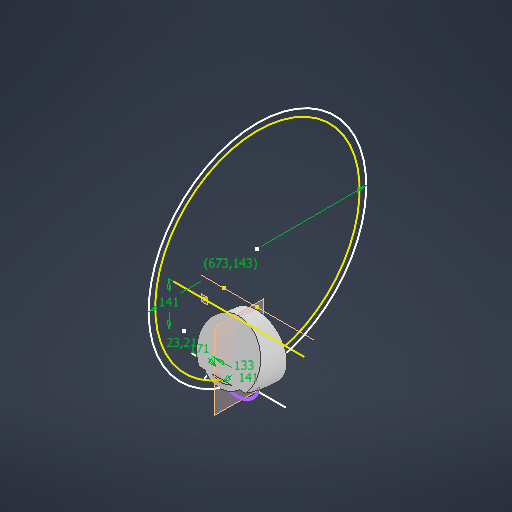
# Autodesk Inventor part: направление мяча 2
Saved by Autodesk Inventor 2026.2 (Build 302298000, 298)
## iProperties
Created: 2025-11-28
Part Number: направление мяча 2
Material: Типовые
Document SubType Name: Modeling
Designer: Phantom
Density: 1 g/cm^3
Appearance: По умолчанию
Author: Phantom
Autodesk Inventor part; units mm, degrees
ref_plane "XZ Plane" through (0, 0, 0) normal (0, 1, 0) x (-1, 0, 0)
sketch "Эскиз1" plane through (0, 0, 0) normal (0, 0, 1) x (1, 0, 0)
  arc A0 (72.3251, -161) -> (129.6749, -161) centre (101, -101) ccw
  arc A1 (47.332, -161) -> (154.668, -161) centre (101, -101) ccw
  line L0 (-97.5257, 0) -> (307.6841, 0) projected
  line L1 (-39.6386, -161) -> (244.9538, -161)
  line L2 (101, -167.5) -> (101, -181.5)
  arc A2 (171.1424, -161) -> (30.8576, -161) centre (101, -101) ccw
  arc A3 (169.1564, -161) -> (32.8436, -161) centre (101, -101) ccw
  arc A4 (173.1049, -161) -> (28.8951, -161) centre (101, -101) ccw
  line L3 (188.8611, -125.2269) -> (188.512, -125.2269)
  line L4 (188.512, -125.2269) -> (191.6745, -125.0262)
  line L5 (13.488, -125.2269) -> (10.3255, -125.0262)
  point P0 (0, 0)
  point P1 (167.5699, -124.21)
  point P2 (163.3181, -124.21)
  point P3 (38.6819, -124.21)
  point P4 (34.4301, -124.21)
  point P5 (101, -174.5)
  point P6 (10.3255, -125.0262)
  point P7 (13.488, -125.2269)
  point P8 (170.7391, -120.21)
  dimension "d0" = 133
  dimension "d1" = 161
  dimension "d3" = -101
  dimension "d4" = 60
  dimension "d30" = 1.5
  dimension "d31" = 1.5
  dimension "d33" = 92.3036
  constraints: 14 point on circle, 8 end point, 5 centre point, 2 coincident, 2 midpoint, 2 symmetric about line, 1 horizontal, 13 other
  measures "d0" diameter of A0
  measures "d1" diameter of A1
  measures "d3" distance from line of A1.centre L0
  measures "d30" radial gap between concentric circles of A2 A3
  measures "d31" radial gap between concentric circles of A2 A4
  measures "d33" radius of A2
ref_plane "РабПлоскость1" through (0, 0, 60) normal (0, 0, 1) x (1, 0, 0)
sketch "Эскиз2" plane through (0, 0, 60) normal (0, 0, 1) x (1, 0, 0)
  circle A0 centre (101, -101) radius 70.5
  line L0 (-96.1046, 0) -> (307.4472, 0) projected
  arc A1 (34.4301, -164.21) -> (167.5699, -164.21) centre (101, -141) ccw
  arc A2 (38.6819, -164.21) -> (163.3181, -164.21) centre (101, -141) ccw
  line L1 (-38.4543, -164.21) -> (249.797, -164.21)
  point P0 (0, 0)
  dimension "d9" = 141
  dimension "d10" = 141
  dimension "d11" = 133
  dimension "d12" = 23.21
  constraints: 4 point on circle, 4 point on line, 3 centre point, 2 end point, 1 coincident, 1 horizontal
  measures "d9" diameter of A1
  measures "d10" distance from line of L0 A1.centre
  measures "d11" diameter of A2
  measures "d12" distance from line of A1.centre L1
sketch "Эскиз3" plane through (0, 0, 0) normal (1, 0, 0) x (0, 1, 0)
  arc A0 (-211.5, 60) -> (-171.5, 0) centre (-52.4181, 122.7213) ccw
  point P0 (0, 0)
  point P1 (-164.21, 60)
  point P2 (-161, 0)
  dimension "d13" = 171
  constraints: 2 point on circle, 1 centre point
  measures "d13" radius of A0
sketch "Эскиз4" plane through (0, 0, 0) normal (1, 0, 0) x (0, 1, 0)
  line L0 (0, -473.8566) -> (0, 468.5441) projected
  arc A0 (-151.3766, 110.2381) -> (-171.5, 0) centre (155.0612, -2.6563) ccw
  arc A1 (-171.3994, 5.874) -> (-171.5, 0) centre (0, 0) ccw
  point P0 (-131.3766, -110.2381)
  dimension "d25" = 326.572
  constraints: 5 point on circle, 2 centre point, 1 coincident
  measures "d25" radius of A0
sweep "Сдвиг2" add profiles "Эскиз1" path "Эскиз4" path curves A0 contours A0 L2 A1 L1 | L1 A3 | A0 L1 A1 L2 | L1 A2 L5 A3 | L1 A4 L5 A2 | L5 A2 L4 A3 | A3 L4 A2 L1 | L5 A4 L4 A2 | A2 L4 A4 L1
ref_plane "РабПлоскость2" through (101, 0, 0) normal (1, 0, 0) x (0, 1, 0)
sketch "Эскиз5" plane through (101, 0, 0) normal (1, 0, 0) x (0, 1, 0)
  line L0 (-161, 0) -> (-161, 0) projected
  arc A0 (-141.4948, 106.6885) -> (-161, 0) centre (155.0612, -2.6563) ccw projected
  line L1 (-141.4948, 106.6885) -> (-141.4948, 106.6885) projected
  arc A1 (-141.4948, 106.6885) -> (-161, 0) centre (155.0612, -2.6563) ccw projected
  line L2 (-161, 0) -> (-161, 0) projected
  arc A2 (-141.4948, 106.6885) -> (-161, 0) centre (155.0612, -2.6563) ccw projected
  line L3 (-141.4948, 106.6885) -> (-141.4948, 106.6885) projected
  arc A3 (-141.4948, 106.6885) -> (-161, 0) centre (155.0612, -2.6563) ccw projected
  arc A4 (-161, 0) -> (-141.4948, 106.6885) centre (155.0612, -2.6563) ccw projected
  line L4 (-161, 0) -> (-181.5, 0) projected
  circle A5 centre (155.0612, -2.6563) radius 336.5717
  point P0 (0, 0)
  dimension "d28" = 673.1434
  constraints: 1 coincident, 3 other
